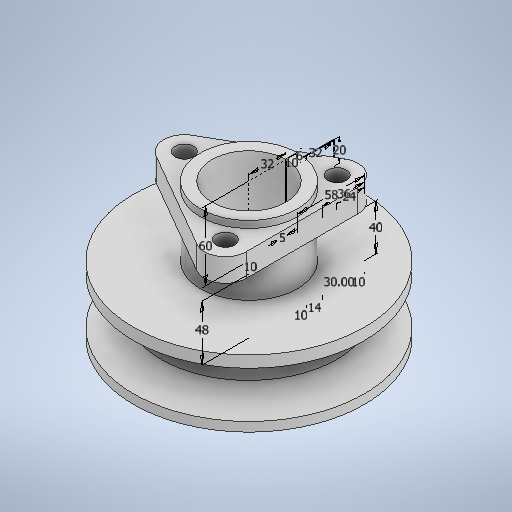
# Autodesk Inventor part: baitap1
Saved by Autodesk Inventor 2025.1 (Build 291241000, 241)
## iProperties
Created: 2024-10-01
Part Number: baitap1
Material: Generic
Document SubType Name: Modeling
Designer: msi
Density: 1 g/cm^3
Appearance: Default
Author: msi
Autodesk Inventor part; units mm, degrees
ref_plane "YZ Plane" through (0, 0, 0) normal (1, 0, 0) x (0, 1, 0)
ref_plane "XZ Plane" through (0, 0, 0) normal (0, 1, 0) x (-1, 0, 0)
ref_plane "XY Plane" through (0, 0, 0) normal (0, 0, 1) x (1, 0, 0)
sketch "Sketch2" plane through (0, 0, 0) normal (1, 0, 0) x (0, 1, 0)
  line L0 (0, 0) -> (48, 0) construction
  line L1 (48, 0) -> (58, 0) construction
  line L2 (58, 0) -> (118, 0) construction
  line L3 (118, 0) -> (118, -32) construction
  line L4 (118, -32) -> (118, -42)
  line L5 (118, -42) -> (112, -42)
  line L6 (112, -42) -> (112, -74)
  line L7 (92, -74) -> (92, -42)
  line L8 (92, -42) -> (58, -42)
  line L9 (58, -42) -> (58, -100)
  line L10 (58, -100) -> (48, -100)
  line L11 (48, -100) -> (8, -100) construction
  line L12 (8, -100) -> (0, -100)
  line L13 (0, -100) -> (0, 0) construction
  line L14 (58, -100) -> (58, -64)
  line L15 (58, -64) -> (0, -64) construction
  line L16 (48, -100) -> (48, 0) construction
  line L17 (0, -64) -> (0, -50) construction
  line L18 (58, -100) -> (58, -76)
  line L19 (58, -76) -> (0, -76) construction
  line L20 (48, -100) -> (34.1436, -76)
  line L21 (8, -100) -> (21.8564, -76)
  line L22 (0, -100) -> (0, -90)
  line L23 (0, -50) -> (48, -50)
  line L24 (0, -90) -> (15.0111, -64)
  line L25 (0, -50) -> (0, -40)
  line L26 (0, -40) -> (48, -40)
  line L27 (48, -64) -> (15.0111, -64)
  line L28 (34.1436, -76) -> (21.8564, -76)
  line L29 (118, -32) -> (48, -32) construction
  line L30 (58, 0) -> (58, -32) construction
  line L31 (58, -32) -> (58, -27)
  line L32 (58, -27) -> (48, -27)
  line L33 (118, -32) -> (58, -32)
  line L34 (48, -27) -> (48, -40)
  line L35 (48, -50) -> (48, -64)
  line L36 (28, -100) -> (28, -76) construction
  line L37 (112, -74) -> (92, -74)
  dimension "d0" = 48
  dimension "d1" = 10
  dimension "d2" = 60
  dimension "d3" = 32
  dimension "d4" = 10
  dimension "d5" = 6
  dimension "d6" = 32
  dimension "d7" = 20
  dimension "d9" = 58
  dimension "d10" = 40
  dimension "d11" = 36
  dimension "d12" = 14
  dimension "d13" = 24
  dimension "d17" = 10
  dimension "d19" = 30
  dimension "d20" = 10
  dimension "d21" = 5
  constraints: 76 end point, 22 point on line, 13 perpendicular, 4 horizontal, 4 midpoint, 3 collinear, 3 parallel, 2 vertical, 1 other
  measures "d0" distance of L0.start L0.end
  measures "d1" distance of L0.end L1.end
  measures "d2" distance of L1.end L2.end
  measures "d3" distance of L2.end L3.end
  measures "d4" distance of L3.end L4.end
  measures "d5" distance of L4.end L5.end
  measures "d6" distance of L5.end L6.end
  measures "d7" distance of L6.end L7.start
  measures "d9" distance of L8.end L9.end
  measures "d10" distance of L10.end L11.end
  measures "d11" distance of L9.end L14.end
  measures "d12" distance of L15.end L17.end
  measures "d13" distance of L9.end L18.end
  measures "d17" distance of L12.end L22.end
  measures "d19" angle of L13 L24
  measures "d20" distance of L17.end L25.end
  measures "d21" distance of L30.end L31.end
revolve "Revolution1" add sketch "Sketch2" angle 360 about axis through (0, 58, 0) along (0, 1, 0)
sketch "Sketch6" plane through (0, 112, 0) normal (0, 1, 0) x (1, 0, 0)
  circle A0 centre (0, 0) radius 56 construction
  circle A1 centre (-56, 0) radius 8
  circle A2 centre (-56, 0) radius 18 construction
  line L0 (-74, 0) -> (74, 0) construction
  circle A3 centre (0, 0) radius 74 projected
  line L1 (-74, 0) -> (37, -64.0859) construction
  line L2 (37, -64.0859) -> (0, 0) construction
  line L3 (-74, 0) -> (37, 64.0859) construction
  line L4 (37, -64.0859) -> (37, 64.0859) construction
  circle A4 centre (28, -48.4974) radius 18 construction
  circle A5 centre (28, -48.4974) radius 8
  line L5 (0, 0) -> (37, 64.0859) construction
  circle A6 centre (28, 48.4974) radius 8
  circle A7 centre (28, 48.4974) radius 18 construction
  line L6 (-65, -15.5885) -> (19, -64.0859)
  line L7 (-64, 16.1245) -> (18.9942, 64.0825)
  line L8 (46, -48.4974) -> (46, 48.4974)
  arc A8 (46, 48.4974) -> (18.9942, 64.0825) centre (28, 48.4974) ccw
  arc A9 (-64, 16.1245) -> (-65, -15.5885) centre (-56, 0) ccw
  arc A10 (19, -64.0859) -> (46, -48.4974) centre (28, -48.4974) ccw
  point P0 (37, -64.0859)
  dimension "d26" = 112
  dimension "d27" = 16
  dimension "d28" = 36
  dimension "d29" = 30
  dimension "d30" = 36
  dimension "d31" = 16
  dimension "d32" = 16
  dimension "d33" = 36
  constraints: 18 end point, 18 point on circle, 10 centre point, 7 coincident, 3 tangent, 2 point on line, 1 horizontal, 1 symmetric about line, 1 vertical
  measures "d26" diameter of A0
  measures "d27" diameter of A1
  measures "d28" diameter of A2
  measures "d29" angle of L0 L1
  measures "d30" diameter of A4
  measures "d31" diameter of A5
  measures "d32" diameter of A6
  measures "d33" diameter of A7
extrude "Extrusion1" cut sketch "Sketch6" against normal blind 20 contours A1 | A3 A10 L8 A8 | A8 L7 A9 A3 | A3 A9 L6 A10 | A5 | A6
body "Solid1"
